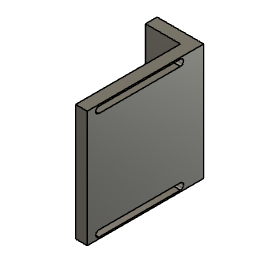
LaserSaftyInterlockOverrideHolder v3 (Autodesk Fusion 360 design; units mm, degrees)
Autodesk Fusion 360 part; units mm, degrees
sketch "Sketch1" plane through (0, 0, 0) normal (0, 0, 1) x (1, 0, 0)
  line L0 (5, 5) -> (-5, 5)
  line L1 (-5, 5) -> (-5, -5)
  line L2 (-5, -5) -> (5, -5)
  line L3 (5, -5) -> (5, 5)
  line L4 (5, 5) -> (-5, -5) construction
  line L5 (-5, 5) -> (5, -5) construction
  line L6 (-5, 5) -> (5, 5)
  line L7 (5, 5) -> (5, 25)
  line L8 (5, 25) -> (-5, 25)
  line L9 (-5, 25) -> (-5, 5)
  circle A0 centre (0, 15) radius 4.5
  line L10 (-5, -15) -> (5, -15) construction
  line L11 (0, 25) -> (0, 5) construction
  line L12 (-5, 15) -> (5, 15) construction
  line L13 (20, 0) -> (2.5, 0) construction
  line L14 (5, -25) -> (-5, -25)
  line L15 (5, -5) -> (5, -25)
  line L16 (-5, -25) -> (-5, -5)
  circle A1 centre (0, -15) radius 4.5
  dimension "d1" = 10
  dimension "d2" = 10
  dimension "d3" = 20
  dimension "d4" = 9
  dimension "d5" = 10
  dimension "d6" = 10
  constraint horizontal L0
  constraint perpendicular L0 L1
  constraint parallel L0 L2
  constraint parallel L1 L3
  constraint coincident L4 origin
  constraint coincident L5 origin
  constraint horizontal L6
  constraint vertical L7
  constraint horizontal L8
  constraint vertical L9
  constraint coincident L9 L10.start
  constraint coincident L7 L10.end
  constraint perpendicular L7 L10
  constraint midpoint L8 L11.start
  constraint midpoint L6 L11.end
  constraint symmetric L0 L8 L10
  constraint coincident L9 L12.start
  constraint coincident L7 L12.end
  constraint perpendicular L7 L12
  constraint coincident A0.centre L12
  constraint coincident A0.centre L11
  constraint symmetric L0.end L13 L1.end
  constraint symmetric L0.start L13 L2.end
  constraint symmetric L7.end L13 L14.start
  constraint symmetric L8.end L13 L14.end
  constraint symmetric A0 L13 A1
  measures "d1" distance of L1.end L2.end
  measures "d2" distance of L0.end L1.end
  measures "d3" distance of L0.end L8.end
  measures "d4" diameter of A0
  measures "d5" distance of L7 L9
  measures "d6" distance of L8 L12
extrude "Extrude1" add sketch "Sketch1" against normal blind 10 contours L0 L1 L2 L3 L6
extrude "Extrude2" add sketch "Sketch1" 1 faces at (-1.6667, -1.6667, 0) along normal blind 10 contours L0 L6 L7 L8 L9 | L2 L14 L15 L16
sketch "Sketch2" plane through (5, 0, 0) normal (1, 0, 0) x (0, 0, -1)
  line L0 (0, -5) -> (10, -5)
  line L1 (10, -5) -> (10, 5)
  line L2 (10, 5) -> (0, 5)
  line L3 (0, 5) -> (0, 25)
  line L4 (0, 25) -> (-10, 25)
  line L5 (-10, 25) -> (-10, -25)
  line L6 (-10, -25) -> (0, -25)
  line L7 (0, -25) -> (0, -5)
  line L8 (-10, 25) -> (0, 25)
  line L9 (0, 25) -> (0, -25)
  line L10 (0, -25) -> (-10, -25)
  line L11 (-10, -25) -> (-10, 25)
  constraint horizontal L8
  constraint vertical L9
  constraint horizontal L10
  constraint vertical L11
  constraint coincident L6.end L7.start
  constraint coincident L4.end L5.start
extrude "Extrude3" add sketch "Sketch2" along normal blind 15 contours L3 L4 L5 L6 L7 L8 L9 L10 L11
sketch "Sketch3" plane through (0, 0, 10) normal (0, 0, 1) x (1, 0, 0)
  circle A0 centre (0, -15) radius 4.5
  circle A1 centre (0, 15) radius 4.5
  line L0 (-5, 25) -> (-5, -25)
  line L1 (-5, -25) -> (20, -25)
  line L2 (20, -25) -> (20, 25)
  line L3 (20, 25) -> (-5, 25)
  line L4 (10, -25) -> (20, -25)
  line L5 (20, 50) -> (10, 50)
  line L6 (10, 50) -> (10, -50)
  line L7 (10, -50) -> (20, -50)
  line L8 (20, -50) -> (20, 50)
  line L9 (20, 50) -> (10, -50) construction
  line L10 (10, 50) -> (20, -50) construction
  line L11 (20, 0) -> (2.5, 0)
  point P0 (15, 0)
  point P1 (20, 0)
  dimension "d29" = 10
  dimension "d30" = 100
  dimension "d31" = 50
  constraint coincident L1 L4.start
  constraint horizontal L5
  constraint perpendicular L5 L6
  constraint parallel L5 L7
  constraint parallel L6 L8
  constraint coincident L9 P0
  constraint coincident L10 P0
  constraint coincident L8 P1
  measures "d29" distance of L6.end L7.end
  measures "d30" distance of L5.end L6.end
  measures "d31" distance of L7 L11
extrude "Extrude4" add sketch "Sketch3" along normal blind 90 contours L3 L5 L6 L8 | L2 L3 L6 L8 L11 | L1 L2 L4 L6 L8 L11 | L1 L4 L6 L7 L8
extrude "Extrude7" add sketch "Sketch3" against normal blind 10 contours L3 L5 L6 L8 | L1 L4 L6 L7 L8
sketch "Sketch4" plane through (20, 0, 0) normal (1, 0, 0) x (0, 0, -1)
  line L0 (0, -50) -> (0, 50)
  line L1 (-100, 50) -> (-100, -50)
  line L2 (-100, 0) -> (0, 0) construction
  circle A0 centre (-90, 46) radius 2.75
  circle A1 centre (-20, 46) radius 2.75
  line L3 (-90, 48.75) -> (-20, 48.75)
  line L4 (-20, 43.25) -> (-90, 43.25)
  line L5 (0, 5) -> (0, 25)
  circle A2 centre (-90, -46) radius 2.75
  line L6 (-90, -48.75) -> (-20, -48.75)
  line L7 (-20, -43.25) -> (-90, -43.25)
  circle A3 centre (-20, -46) radius 2.75
  line L8 (0, 50) -> (-100, 50)
  line L9 (-100, -50) -> (0, -50)
  dimension "d15" = 5.5
  dimension "d16" = 5.5
  dimension "d17" = 46
  dimension "d24" = 70
  dimension "d25" = 10
  constraint midpoint L1 L2.start
  constraint coincident L2.end origin
  constraint coincident A0 L3.start
  constraint coincident A1 L3.end
  constraint tangent A1 L3
  constraint coincident A1 L4.start
  constraint coincident A0 L4.end
  constraint tangent A0 L4
  constraint horizontal L4
  constraint tangent A1 L4
  constraint tangent A0 L3
  constraint parallel L3 L4
  constraint symmetric L2 A0 A2
  constraint symmetric L2 A1 A3
  constraint symmetric L2 L3.start L6.start
  constraint symmetric L2 L3.end L6.end
  constraint symmetric L2 L4.start L7.start
  constraint symmetric L2 L4.end L7.end
  measures "d15" diameter of A0
  measures "d16" diameter of A1
  measures "d17" distance of L2 A1.centre
  measures "d24" distance of A0.centre A1.centre
  measures "d25" distance of L1 A0.centre
extrude "Extrude5" cut sketch "Sketch4" against normal through all contours A0 | A0 A1 L3 L4 | A1 | A2 | A2 L6 L7 A3 | A3
sketch "Sketch5" plane through (-5, 0, 0) normal (-1, 0, 0) x (0, 0, 1)
  line L0 (0, 5) -> (-10, 5)
  line L1 (-10, 5) -> (-10, -5)
  line L2 (-10, -5) -> (0, -5)
  line L3 (0, -5) -> (0, -25)
  line L4 (0, -25) -> (10, -25)
  line L5 (10, 25) -> (0, 25)
  line L6 (0, 25) -> (0, 5)
  line L7 (0, 25) -> (10, 25)
  line L8 (10, 25) -> (10, -25)
  line L9 (10, -25) -> (0, -25)
  line L10 (0, -25) -> (0, 25)
  line L11 (10, -25) -> (10, 25)
  constraint horizontal L7
  constraint vertical L8
  constraint horizontal L9
  constraint vertical L10
  constraint coincident L4.end L8.end
  constraint coincident L5.end L6.start
sketch "Sketch7" plane through (-5, 0, 0) normal (-1, 0, 0) x (0, 0, 1)
  line L0 (0, 5) -> (-10, 5)
  line L1 (-10, 5) -> (-10, -5)
  line L2 (-10, -5) -> (0, -5)
  line L3 (0, -5) -> (0, -25)
  line L4 (0, -25) -> (10, -25)
  line L5 (10, -25) -> (10, 25)
  line L6 (10, 25) -> (0, 25)
  line L7 (0, 25) -> (0, 5)
  line L8 (0, 50) -> (10, 50)
  line L9 (10, 50) -> (10, -50)
  line L10 (10, -50) -> (0, -50)
  line L11 (0, -50) -> (0, 50)
  constraint horizontal L8
  constraint vertical L9
  constraint horizontal L10
  constraint vertical L11
extrude "Extrude9" add sketch "Sketch7" along normal blind 15 contours L3 L4 L5 L6 L7 L9 L11 | L6 L8 L9 L11 | L4 L9 L10 L11
extrude "Extrude10" add 2 faces at (-5, 41.6667, 6.6667) (-5, -41.6667, 6.6667) along direction (1, 0, 0) blind 15
equation "d17 = ( 92 / 2 ) * 1 mm"
